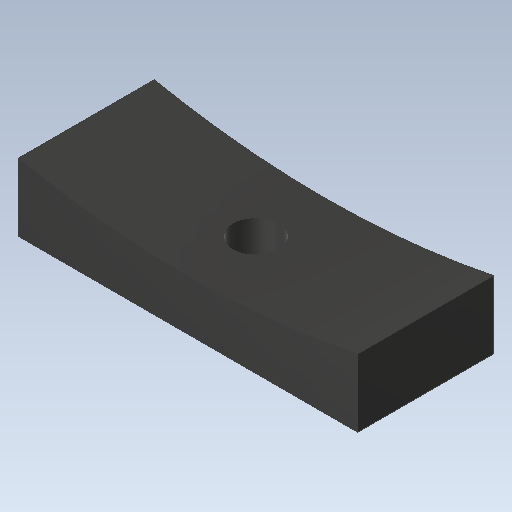
# Autodesk Inventor part: podkladka
Saved by Autodesk Inventor 2020 (Build 240168000, 168)
## iProperties
Created: 2019-06-01
Part Number: podkladka
Material: ABS Plastic
Document SubType Name: Modeling
Designer: Esterka
Density: 1.06 g/cm^3
Appearance: Smooth - White
Author: Esterka
Autodesk Inventor part; units mm, degrees
ref_plane "YZ Plane" through (0, 0, 0) normal (1, 0, 0) x (0, 1, 0)
ref_plane "XZ Plane" through (0, 0, 0) normal (0, 1, 0) x (-1, 0, 0)
ref_plane "XY Plane" through (0, 0, 0) normal (0, 0, 1) x (1, 0, 0)
sketch "Sketch1" plane through (0, 0, 0) normal (0, 0, 1) x (1, 0, 0)
  line L0 (-7.5692, 0) -> (42.4308, 0)
  line L1 (42.4308, 0) -> (42.4308, 10)
  line L2 (-7.5692, 0) -> (-7.5692, 10)
  arc A0 (-7.5692, 10) -> (42.4308, 10) centre (17.4308, 132.4745) ccw
  point P0 (0, 0)
  dimension "d1" = 50
  dimension "d2" = 10
  dimension "d3" = 10
  dimension "d4" = 250
  constraints: 6 end point, 2 point on circle, 1 centre point, 1 horizontal, 1 perpendicular, 1 vertical
  measures "d1" distance of L0.start L0.end
  measures "d2" distance of L0.end L1.end
  measures "d3" distance of L0.start L2.end
  measures "d4" diameter of A0
extrude "Extrusion1" add sketch "Sketch1" along normal blind 20
sketch "Sketch2" plane through (-7.5692, 0, 0) normal (0, -1, 0) x (1, 0, 0)
  line L0 (0, 0) -> (50, 0) projected
  point P0 (7.5692, 0)
  point P1 (25, 10)
  dimension "d7" = 10
  measures "d7" distance from line of L0 point (25, 10)
hole "Hole1" at (17.4308, 0, 10) direction (0, 1, 0) diameter 6.756 end through all clearance for "Flat Head Machine Screw (82)" size "1/4" standard "Ansi Unified Screw Threads"
body "Solid1"
